Autodesk Fusion 360 part; units mm, degrees
(part 2 of 2)
equation "d39 = d40 + ( 8 / 15 ) * 1 mm"
equation "d53 = -d23"
equation "d64 = d61"
equation "d67 = d61"
equation "d88 = d86"
equation "d89 = d86"
equation "d92 = d90"
equation "d93 = d90"
equation "d96 = d94"
equation "d97 = d94"
equation "d100 = d94"
equation "d102 = d94"
equation "d108 = d107"
equation "d109 = d107"
equation "d110 = d107"
equation "d112 = d111"
equation "d120 = d119"
equation "d124 = d123"
equation "d142 = d51"
equation "d150 = d149"
equation "d151 = d149"
equation "d153 = d152"
equation "d154 = d152"
